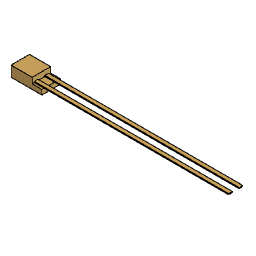
MC Lid assembly laser v9 (Autodesk Fusion 360 archive; units mm, degrees)
design "Lakeshore DT 670 SD Omega CY 670 SD"
Autodesk Fusion 360 part; units mm, degrees
sketch "Sketch1" plane through (0, 0, 0) normal (0, 0, 1) x (1, 0, 0)
  line L0 (0, 0) -> (3.175, 0)
  line L1 (3.175, 0) -> (3.175, 0.5)
  line L2 (3.175, 0.5) -> (2.175, 0.5)
  line L3 (2.175, 0.5) -> (2.175, 1.08)
  line L4 (2.175, 1.08) -> (0, 1.08)
  line L5 (0, 1.08) -> (0, 0)
  dimension "d1" = 1.08
  dimension "d2" = 3.175
  dimension "d3" = 1
  dimension "d4" = 0.5
  constraint coincident L0.start L5.end
  constraint horizontal L0
  constraint perpendicular L0 L1
  constraint perpendicular L1 L2
  constraint perpendicular L0 L3
  constraint perpendicular L3 L4
  constraint perpendicular L0 L5
  measures "d1" distance of L4.end L0.start
  measures "d2" distance of L0.start L0.end
  measures "d3" distance of L1.end L2.end
  measures "d4" distance of L0.end L1.end
extrude "Extrude1" add sketch "Sketch1" along normal blind 1.905
sketch "Sketch2" plane through (0, 0.5, 0) normal (0, 1, 0) x (-1, 0, 0)
  line L0 (-3.175, 0) -> (-2.175, 0)
  line L1 (-2.175, 0) -> (-2.175, 1.905)
  line L2 (-2.175, 1.905) -> (-3.175, 1.905)
  line L3 (-3.175, 1.905) -> (-3.175, 0)
  line L4 (-2.175, 0.2225) -> (-22.175, 0.2225)
  line L5 (-22.175, 0.2225) -> (-22.175, 0.6035)
  line L6 (-22.175, 0.6035) -> (-2.175, 0.6035)
  line L7 (-2.175, 0.6035) -> (-2.175, 0.2225)
  line L8 (-3.175, 0.9525) -> (0, 0.9525) construction
  line L9 (-2.175, 1.6825) -> (-22.175, 1.6825)
  line L10 (-22.175, 1.3015) -> (-2.175, 1.3015)
  line L11 (-22.175, 1.6825) -> (-22.175, 1.3015)
  line L12 (-2.175, 1.3015) -> (-2.175, 1.6825)
  dimension "d7" = 0.381
  dimension "d8" = 19
  dimension "d9" = 0.698
  constraint horizontal L4
  constraint vertical L5
  constraint horizontal L6
  constraint vertical L7
  constraint collinear L1 L7
  constraint midpoint L3 L8.start
  constraint perpendicular L3 L8
  constraint symmetric L4.start L8 L9.start
  constraint symmetric L4.end L8 L9.end
  constraint symmetric L5.end L8 L10.start
  constraint symmetric L6.end L8 L10.end
  measures "d7" distance of L4.end L5.end
  measures "d8" distance of L3 L5
  measures "d9" distance of L6 L10
extrude "Extrude2" add sketch "Sketch2" along normal blind 0.102 contours L3 L4 L5 L6 | L1 L3 L4 L6 L7 | L3 L9 L10 L11 | L1 L3 L9 L10 L12

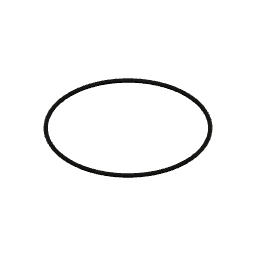
design "O ring 145 x 4"
Autodesk Fusion 360 part; units mm, degrees
sketch "Sketch1" plane through (0, 0, 0) normal (0, 0, 1) x (1, 0, 0)
  circle A0 centre (74.5, 0) radius 2
  dimension "d1" = 4
  dimension "d2" = 74.5
  constraint horizontal origin A0.centre
  measures "d1" diameter of A0
  measures "d2" horizontal distance of origin A0.centre
revolve "Revolve1" add sketch "Sketch1" angle 360 about axis through (0, 1.75, 0) along (0, 1, 0)
equation "d2 = ( 145 / 2 ) * 1 mm + 2 mm"

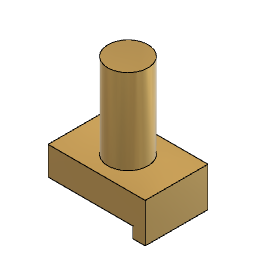
design "Lakeshore CO clamp"
Autodesk Fusion 360 part; units mm, degrees
sketch "Sketch1" plane through (0, 0, 0) normal (0, 0, 1) x (1, 0, 0)
  line L0 (0, 0) -> (0, 3.2)
  line L1 (0, 3.2) -> (-7.9, 3.2)
  line L2 (-7.9, 3.2) -> (-7.9, 0.9)
  line L3 (-7.9, 0.9) -> (-1, 0.9)
  line L4 (-1, 0.9) -> (-1, 0)
  line L5 (-1, 0) -> (0, 0)
  dimension "d1" = 3.2
  dimension "d2" = 7.9
  dimension "d3" = 0.9
  dimension "d4" = 1
  constraint coincident L0.start L5.end
  constraint vertical L0
  constraint perpendicular L0 L1
  constraint perpendicular L1 L2
  constraint perpendicular L2 L3
  constraint perpendicular L1 L4
  constraint perpendicular L0 L5
  measures "d1" distance of L0.start L0.end
  measures "d2" distance of L0.end L1.end
  measures "d3" distance of L3.end L4.end
  measures "d4" distance of L4.end L0.start
extrude "Extrude1" add sketch "Sketch1" along normal blind 5.1
hole "Hole1" at (-3.95, 3.2, 2.55) direction (0, -1, 0) diameter 3.264 depth 5 tip angle 118
sketch "Sketch2" plane through (0, 0, 0) normal (0, 1, 0) x (1, 0, 0)
  circle A0 centre (-3.95, -2.55) radius 2
  circle A1 centre (-3.95, -2.55) radius 1.632
  dimension "d10" = 4
  constraint concentric A0 A1
  measures "d10" diameter of A0
extrude "Extrude2" add sketch "Sketch2" along normal up to surface (10.1 mm away) contours A1
